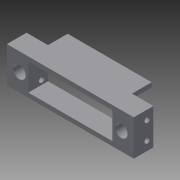
# Autodesk Inventor part: tendeur_base_low
Saved by Autodesk Inventor 2014 SP1 (Build 180222100, 222)
## iProperties
Created: 2015-09-12
Part Number: tendeur_base_low
Material: Générique
Document SubType Name: Modeling
Designer: astralien3000
Density: 1 g/cm^3
Appearance: Par défaut
Author: astralien3000
Autodesk Inventor part; units mm, degrees
ref_plane "YZ Plane" through (0, 0, 0) normal (1, 0, 0) x (0, 1, 0)
ref_plane "XZ Plane" through (0, 0, 0) normal (0, 1, 0) x (-1, 0, 0)
ref_plane "XY Plane" through (0, 0, 0) normal (0, 0, 1) x (1, 0, 0)
sketch "Esquisse1" plane through (0, 0, 0) normal (0, 1, 0) x (-1, 0, 0)
  circle A0 centre (-28.5, 0) radius 3.5
  circle A1 centre (28.5, 0) radius 3.5
  line L0 (-35.5, 10) -> (35.5, 10)
  line L1 (35.5, 10) -> (35.5, -10)
  line L2 (35.5, -10) -> (-35.5, -10)
  line L3 (-35.5, -10) -> (-35.5, 10)
  line L4 (-28.5, 0) -> (28.5, 0)
  point P0 (0, 0)
  dimension "d0" = 7
  dimension "d1" = 7
  dimension "d2" = 28.5
  dimension "d3" = 28.5
  dimension "d4" = 20
  dimension "d5" = 10
  dimension "d6" = 7
  dimension "d7" = 7
  constraints: 10 end point, 2 centre point, 2 parallel, 2 perpendicular, 1 horizontal, 1 midpoint
  measures "d0" diameter of A0
  measures "d1" diameter of A1
  measures "d2" distance of L4.end point (0, 0)
  measures "d3" distance of point (0, 0) L4.start
  measures "d4" distance between parallel lines of L2 L0
  measures "d5" distance from line of L0 L4.end
  measures "d6" distance from line of L1 L4.end
  measures "d7" distance from line of L3 L4.start
extrude "Extrusion1" add sketch "Esquisse1" along normal blind 22
sketch "Esquisse2" plane through (0, 22, 0) normal (0, 1, 0) x (1, 0, 0)
  circle A0 centre (-28.5, 0) radius 3.5 projected
  circle A1 centre (28.5, 0) radius 3.5 projected
  line L0 (-23.5, 7.5) -> (23.5, 7.5)
  line L1 (23.5, 7.5) -> (23.5, -7.5)
  line L2 (23.5, -7.5) -> (-23.5, -7.5)
  line L3 (-23.5, -7.5) -> (-23.5, 7.5)
  point P0 (0, 0)
  dimension "d10" = 15
  dimension "d11" = 7.5
  dimension "d12" = 5
  dimension "d13" = 5
  constraints: 8 end point, 2 parallel, 1 horizontal, 1 perpendicular
  measures "d10" distance between parallel lines of L2 L0
  measures "d11" distance from line of point (0, 0) L0
  measures "d12" distance from line of L1 A1.centre
  measures "d13" distance from line of A0.centre L3
extrude "Extrusion2" cut sketch "Esquisse2" against normal through all contours L0 L1 L2 L3
sketch "Esquisse3" plane through (-35.5, 0, 10) normal (0, 0, 1) x (1, 0, 0)
  line L0 (71, 0) -> (0, 0) projected
  line L1 (71, 0) -> (71, 22) projected
  line L2 (0, 22) -> (71, 22) projected
  line L3 (0, 0) -> (0, 22) projected
  line L4 (14, 22) -> (57, 22)
  line L5 (57, 22) -> (57, 0)
  line L6 (57, 0) -> (14, 0)
  line L7 (14, 0) -> (14, 22)
  line L8 (14, 22) -> (22, 22)
  line L9 (22, 22) -> (22, 14)
  line L10 (22, 14) -> (14, 14)
  line L11 (14, 14) -> (14, 22)
  line L12 (57, 22) -> (49, 22)
  line L13 (49, 22) -> (49, 14)
  line L14 (49, 14) -> (57, 14)
  line L15 (57, 14) -> (57, 22)
  line L16 (14, 22) -> (22, 14)
  line L17 (22, 22) -> (14, 14)
  line L18 (49, 14) -> (57, 22)
  line L19 (49, 22) -> (57, 14)
  circle A0 centre (18, 18) radius 2
  circle A1 centre (53, 18) radius 2
  point P0 (35.5, 0)
  dimension "d16" = 14
  dimension "d17" = 14
  dimension "d18" = 8
  dimension "d19" = 8
  dimension "d20" = 8
  dimension "d21" = 8
  dimension "d22" = 4
  dimension "d23" = 4
  constraints: 32 end point, 6 parallel, 4 midpoint, 3 horizontal, 3 perpendicular, 2 centre point, 2 point on line
  measures "d16" distance between parallel lines of L1 L5
  measures "d17" distance between parallel lines of L3 L7
  measures "d18" distance of L8.end L9.end
  measures "d19" distance of L9.end L10.end
  measures "d20" distance of L13.end L14.end
  measures "d21" distance of L12.end L13.end
  measures "d22" diameter of A0
  measures "d23" diameter of A1
extrude "Extrusion3" add sketch "Esquisse3" along normal through all both and the other way through all contours A1 L18 L19 | L19 L18 A1 | L18 L19 A1 | A0 L16 L17 | L17 L16 A0 | A1 L19 L18 | A0 L17 L16 | L16 L17 A0
sketch "Esquisse4" plane through (35.5, 0, 10) normal (1, 0, 0) x (0, 0, -1)
  line L0 (20, 0) -> (0, 0) projected
  line L1 (0, 22) -> (20, 22) projected
  line L2 (6.5, 22) -> (13.5, 22)
  line L3 (13.5, 22) -> (13.5, 0)
  line L4 (13.5, 0) -> (6.5, 0)
  line L5 (6.5, 0) -> (6.5, 22)
  circle A0 centre (5, 7.5) radius 1.5
  circle A1 centre (15, 7.5) radius 1.5
  line L6 (20, 0) -> (20, 22) projected
  line L7 (0, 0) -> (6.5, 0)
  line L8 (6.5, 0) -> (6.5, 15)
  line L9 (6.5, 15) -> (0, 15)
  line L10 (0, 15) -> (0, 0)
  line L11 (13.5, 0) -> (20, 0)
  line L12 (20, 0) -> (20, 15)
  line L13 (20, 15) -> (13.5, 15)
  line L14 (13.5, 15) -> (13.5, 0)
  line L15 (0, 0) -> (0, 22) projected
  line L16 (13.5, 7.5) -> (20, 7.5)
  line L17 (0, 7.5) -> (6.5, 7.5)
  point P0 (10, 0)
  dimension "d26" = 7
  dimension "d27" = 3.5
  dimension "d28" = 3
  dimension "d29" = 3
  dimension "d32" = 15
  constraints: 28 end point, 6 parallel, 6 point on line, 4 midpoint, 3 horizontal, 3 perpendicular, 2 centre point, 2 coincident, 2 collinear, 2 tangent
  measures "d26" distance between parallel lines of L5 L3
  measures "d27" distance from line of L3 point (10, 0)
  measures "d28" diameter of A0
  measures "d29" diameter of A1
  measures "d32" distance between parallel lines of L0 L9
extrude "Extrusion4" cut sketch "Esquisse4" against normal through all contours L16 A1 | A1 L16 | L17 A0 | A0 L17
sketch "Esquisse5" plane through (-35.5, 0, 10) normal (0, 0, 1) x (1, 0, 0)
  line L0 (71, 0) -> (0, 0) projected
  line L1 (71, 0) -> (71, 22) projected
  line L2 (0, 22) -> (71, 22) projected
  line L3 (0, 0) -> (0, 22) projected
  line L4 (0, 0) -> (71, 0)
  line L5 (71, 0) -> (71, 11)
  line L6 (71, 11) -> (0, 11)
  line L7 (0, 11) -> (0, 0)
  point P0 (35.5, 0)
  dimension "d33" = 11
  dimension "d34" = 22
  constraints: 8 end point, 2 parallel, 1 horizontal, 1 midpoint, 1 perpendicular
  measures "d33" distance of L6.end L0.end
  measures "d34" distance between parallel lines of L0 L2
extrude "Extrusion5" cut sketch "Esquisse5" against normal through all contours L6 L3 L2 L1
sketch "Esquisse6" plane through (-35.5, 11, 10) normal (0, 1, 0) x (1, 0, 0)
  line L0 (71, 0) -> (0, 0) projected
  line L1 (59, 2.5) -> (59, 17.5) projected
  line L2 (12, 2.5) -> (59, 2.5)
  line L3 (59, 2.5) -> (59, 0)
  line L4 (59, 0) -> (12, 0)
  line L5 (12, 0) -> (12, 2.5)
  point P0 (35.5, 10)
  constraints: 8 end point, 2 parallel, 1 collinear, 1 horizontal, 1 perpendicular, 1 point on line
extrude "Extrusion6" add sketch "Esquisse6" along normal blind 11
equation "\"d3\" = d2"
equation "\"d5\" = 0.5 * d4"
equation "\"d11\" = 0.5 * d10"
equation "\"d17\" = d16"
equation "\"d27\" = 0.5 * d26"
